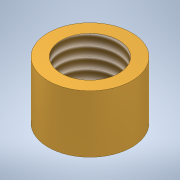
# Autodesk Inventor part: インサートナットM4_4mm_D5.8
Saved by Autodesk Inventor 2022 (Build 260153000, 153)
## iProperties
Created: 2020-10-10
Part Number: インサートナットM4_4mm_D5.8
Material: 真鍮、ソフト イエロー
Document SubType Name: Modeling
Designer: yuta2
Density: 8.47 g/cm^3
Appearance: 真鍮 - サテン
Author: yuta2
Autodesk Inventor part; units mm, degrees
ref_plane "YZ Plane" through (0, 0, 0) normal (1, 0, 0) x (0, 1, 0)
ref_plane "XZ Plane" through (0, 0, 0) normal (0, 1, 0) x (-1, 0, 0)
ref_plane "XY Plane" through (0, 0, 0) normal (0, 0, 1) x (1, 0, 0)
sketch "スケッチ1" plane through (0, 0, 0) normal (0, 1, 0) x (-1, 0, 0)
  circle A0 centre (0, 0) radius 2
  circle A1 centre (0, 0) radius 2.9
  dimension "d0" = 4
  dimension "d1" = 5.8
  constraints: 2 centre point, 2 coincident
  measures "d0" diameter of A0
  measures "d1" diameter of A1
extrude "押し出し1" add sketch "スケッチ1" along normal blind 4
thread "ねじ1" size "M4x0.7" class "6H" standard "ANSI Metric M Profile" full length
